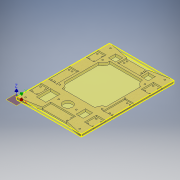
# Autodesk Inventor part: 3枚目
Saved by Autodesk Inventor 2018 (Build 220112000, 112)
## iProperties
Created: 2018-08-16
Part Number: 3枚目
Material: MDF 中密度繊維ボード
Document SubType Name: Modeling
Designer: shun2
Density: 0.8 g/cm^3
Appearance: ダンボール - 段ボール紙
Author: shun2
Autodesk Inventor part; units mm, degrees
ref_plane "YZ Plane" through (0, 0, 0) normal (1, 0, 0) x (0, 1, 0)
ref_plane "XZ Plane" through (0, 0, 0) normal (0, 1, 0) x (-1, 0, 0)
ref_plane "XY Plane" through (0, 0, 0) normal (0, 0, 1) x (1, 0, 0)
ref_plane "作業平面1" through (0, 0, 5.5) normal (0, 0, 1) x (1, 0, 0)
ref_plane "作業平面6" through (0, 0, 5.5) normal (0, 0, 1) x (1, 0, 0)
ref_plane "作業平面7" through (0, 0, 5.5) normal (0, 0, -1) x (-1, 0, 0)
sketch "スケッチ9" plane through (0, 0, 5.5) normal (0, 0, -1) x (-1, 0, 0)
  circle A0 centre (-11, 186.7239) radius 1.6
  circle A1 centre (-11, 8) radius 1.6
  line L0 (-6.4, 186.7239) -> (-15.6, 186.7239)
  line L1 (-6.4, 8) -> (-15.6, 8)
  line L2 (-98, 8) -> (-133, 0)
  line L3 (-46.1667, 8) -> (-3, 0)
  line L4 (0, 0) -> (-3, 0)
  line L5 (-3.0456, 195.0736) -> (-45.187, 186.7239)
  line L6 (-132.9544, 195.0736) -> (-90.813, 186.7239)
  line L7 (-129.6, 186.7239) -> (-120.4, 186.7239)
  circle A2 centre (-125, 186.7239) radius 1.6
  line L8 (-129.6, 8) -> (-120.4, 8)
  circle A3 centre (-125, 8) radius 1.6
  line L9 (-133, 0) -> (-136, 0)
  line L10 (0, 195.0736) -> (-3.0456, 195.0736)
  line L11 (-132.9544, 195.0736) -> (-136, 195.0736)
  line L12 (0, 195.0736) -> (0, 0)
  line L13 (-136, 0) -> (-136, 195.0736)
  line L14 (-90.813, 186.7239) -> (-45.187, 186.7239)
  line L15 (-98, 8) -> (-46.1667, 8)
  point P0 (0, 0)
  constraints: 32 end point, 4 centre point, 4 horizontal, 2 parallel, 1 perpendicular, 1 vertical
extrude "押し出し9" add sketch "スケッチ9" against normal blind 5.5
ref_plane "作業平面8" through (0, 0, 5.5) normal (0, 0, -1) x (-1, 0, 0)
sketch "スケッチ10" plane through (0, 0, 5.5) normal (0, 0, -1) x (-1, 0, 0)
  line L0 (0, 0) -> (0, 225.6064) construction
  circle A0 centre (-68, 39.7463) radius 10
  dimension "d399" = 20
  constraints: 2 end point, 1 centre point, 1 vertical, 1 other
  measures "d399" diameter of A0
extrude "押し出し10" cut sketch "スケッチ10" against normal blind 5.5
sketch "スケッチ13" plane through (0, 0, 11) normal (0, 0, 1) x (1, 0, 0)
  line L0 (117, 65.5) -> (117, 111.126)
  line L1 (117, 65.5) -> (136, 65.5)
  line L2 (136, 111.126) -> (136, 65.5)
  line L3 (117, 111.126) -> (136, 111.126)
  line L4 (19, 65.5) -> (19, 111.126)
  line L5 (19, 65.5) -> (0, 65.5)
  line L6 (0, 111.126) -> (0, 65.5)
  line L7 (19, 111.126) -> (0, 111.126)
  line L8 (0, 40.5) -> (18.3, 40.5) projected
  line L9 (117.7, 40.5) -> (136, 40.5) projected
  line L10 (90.813, 186.7239) -> (45.187, 186.7239) projected
  line L11 (45.187, 186.7239) -> (90.813, 186.7239)
  line L12 (90.813, 186.7239) -> (90.813, 167.7239)
  line L13 (90.813, 167.7239) -> (45.187, 167.7239)
  line L14 (45.187, 167.7239) -> (45.187, 186.7239)
  line L15 (136, 0) -> (136, 195.0736) projected
  line L16 (0, 195.0736) -> (0, 0) projected
  point P0 (105.9625, 75.6175)
  point P1 (244.1196, 130.8174)
  point P2 (0, 62.936)
  point P3 (121.3594, 75.6175)
  point P4 (30.0375, 75.6175)
  point P5 (14.6406, 75.6175)
  dimension "d207" = 45.626
  dimension "d297" = 19
  dimension "d299" = 45.626
  dimension "d300" = 19
  dimension "d394" = 25
  dimension "d395" = 25
  dimension "d428" = 19
  dimension "d458" = 45.626
  constraints: 24 end point, 2 collinear, 2 parallel, 1 horizontal, 1 perpendicular
  measures "d207" distance between parallel lines of L3 L1
  measures "d297" distance between parallel lines of L0 L2
  measures "d299" distance between parallel lines of L7 L5
  measures "d300" distance between parallel lines of L6 L4
  measures "d394" distance between parallel lines of L5 L8
  measures "d395" distance between parallel lines of L1 L9
  measures "d428" distance of L11.end L12.end
  measures "d458" distance between parallel lines of L14 L12
extrude "押し出し13" cut sketch "スケッチ13" against normal blind 2.5
sketch "スケッチ14" plane through (132, 67.436, 11) normal (0, 0, 1) x (1, 0, 0)
  circle A0 centre (0, 39.19) radius 1.6
  line L0 (-15, 43.69) -> (4, 43.69) projected
  circle A1 centre (-6, 39.19) radius 1.6
  circle A2 centre (-6, 2.564) radius 1.6
  line L1 (4, -1.936) -> (-15, -1.936) projected
  circle A3 centre (0, 2.564) radius 1.6
  line L2 (-132, -18.936) -> (-132, 78.7879) projected
  line L3 (-132, 60.7739) -> (4.0811, 60.7739)
  line L4 (4.0811, 60.7739) -> (-63.9594, 60.7739)
  line L5 (-63.9594, 60.7739) -> (-63.9594, 40.19)
  circle A4 centre (-127.9189, 39.19) radius 1.6
  circle A5 centre (-121.9189, 39.19) radius 1.6
  circle A6 centre (-121.9189, 2.564) radius 1.6
  circle A7 centre (-127.9189, 2.564) radius 1.6
  line L6 (4, 28.69) -> (4, -16.936) projected
  circle A8 centre (-82.313, 115.288) radius 1.6
  line L7 (-86.813, 100.2879) -> (-86.813, 119.2879) projected
  circle A9 centre (-82.313, 109.288) radius 1.6
  circle A10 centre (-45.687, 115.288) radius 1.6
  line L8 (-41.187, 119.2879) -> (-41.187, 100.2879) projected
  circle A11 centre (-45.687, 109.288) radius 1.6
  point P0 (-132.5, -84.3342)
  dimension "d261" = 3.2
  dimension "d263" = 4.5
  dimension "d264" = 3.2
  dimension "d266" = 3.2
  dimension "d268" = 4.5
  dimension "d269" = 3.2
  dimension "d309" = 6
  dimension "d310" = 6
  dimension "d311" = 4
  dimension "d312" = 4
  dimension "d322" = 4.5
  dimension "d451" = 3.2
  dimension "d452" = 4.5
  dimension "d453" = 3.2
  dimension "d454" = 6
  dimension "d455" = 3.2
  dimension "d456" = 4.5
  dimension "d457" = 3.2
  constraints: 12 centre point, 6 end point, 4 symmetric about line, 1 horizontal, 1 midpoint, 1 point on line, 1 vertical, 6 other
  measures "d261" diameter of A0
  measures "d264" diameter of A1
  measures "d266" diameter of A2
  measures "d269" diameter of A3
  measures "d309" distance of A2.centre A3.centre
  measures "d310" distance of A1.centre A0.centre
  measures "d311" distance from line of L6 A3.centre
  measures "d312" distance from line of L6 A0.centre
  measures "d451" diameter of A8
  measures "d452" distance from line of L7 A8.centre
  measures "d453" diameter of A9
  measures "d454" distance of A8.centre A9.centre
  measures "d455" diameter of A10
  measures "d456" distance from line of A10.centre L8
  measures "d457" diameter of A11
extrude "押し出し14" cut sketch "スケッチ14" against normal blind 5.5
sketch "スケッチ15" plane through (0, 0, 5.5) normal (0, 0, -1) x (-1, 0, 0)
  circle A0 centre (-86.313, 182.724) radius 1.6 projected
  circle A1 centre (-49.687, 182.724) radius 1.6 projected
  circle A2 centre (-10.0811, 106.626) radius 1.6 projected
  circle A3 centre (-10.0811, 70) radius 1.6 projected
  circle A4 centre (-126, 70) radius 1.6 projected
  circle A5 centre (-132, 106.626) radius 1.6 projected
  circle A6 centre (-126, 106.626) radius 1.6 projected
  circle A7 centre (-132, 70) radius 1.6 projected
  circle A8 centre (-4.0811, 70) radius 1.6 projected
  circle A9 centre (-4.0811, 106.626) radius 1.6 projected
  circle A10 centre (-49.687, 176.724) radius 1.6 projected
  circle A11 centre (-86.313, 176.724) radius 1.6 projected
  circle A12 centre (-68, 39.7463) radius 10 projected
  circle A13 centre (-125, 186.7239) radius 1.6 projected
  circle A14 centre (-125, 8) radius 1.6 projected
  circle A15 centre (-11, 8) radius 1.6 projected
  circle A16 centre (-11, 186.7239) radius 1.6 projected
  line L0 (0, 0) -> (-3, 0) projected
  line L1 (0, 195.0736) -> (0, 0) projected
  line L2 (-3.0456, 195.0736) -> (0, 195.0736) projected
  line L3 (-45.187, 186.7239) -> (-3.0456, 195.0736) projected
  line L4 (-90.813, 186.7239) -> (-45.187, 186.7239) projected
  line L5 (-132.9544, 195.0736) -> (-90.813, 186.7239) projected
  line L6 (-136, 195.0736) -> (-132.9544, 195.0736) projected
  line L7 (-136, 0) -> (-136, 195.0736) projected
  line L8 (-133, 0) -> (-136, 0) projected
  line L9 (-98, 8) -> (-133, 0) projected
  line L10 (-46.1667, 8) -> (-98, 8) projected
  line L11 (-3, 0) -> (-46.1667, 8) projected
  line L12 (-68, 157.5716) -> (-68, 90.4161)
  circle A17 centre (-23.55, 157.5716) radius 1.6
  circle A18 centre (-23.55, 67.4016) radius 1.6
  line L13 (-33.55, 162.5716) -> (-68, 162.5716)
  line L14 (-33.55, 62.4016) -> (-68, 62.4016)
  arc A19 (-33.55, 162.5716) -> (-23.55, 148.4295) centre (-18.55, 162.5716) ccw
  arc A20 (-4.9029, 68.6272) -> (-5.6778, 70.1028) centre (-18.55, 62.4016) ccw
  arc A21 (-23.55, 76.5438) -> (-33.55, 62.4016) centre (-18.55, 62.4016) ccw
  line L15 (-23.55, 148.4295) -> (-23.55, 76.5438)
  circle A22 centre (-112.45, 157.5716) radius 1.6
  circle A23 centre (-112.45, 67.4016) radius 1.6
  line L16 (-102.45, 162.5716) -> (-68, 162.5716)
  line L17 (-102.45, 62.4016) -> (-68, 62.4016)
  arc A24 (-112.45, 148.4295) -> (-102.45, 162.5716) centre (-117.45, 162.5716) ccw
  arc A25 (-102.45, 62.4016) -> (-112.45, 76.5438) centre (-117.45, 62.4016) ccw
  line L18 (-112.45, 148.4295) -> (-112.45, 76.5438)
  constraints: 14 end point, 12 point on circle, 9 centre point, 8 symmetric about line, 1 perpendicular, 1 vertical, 4 other
extrude "押し出し16" cut sketch "スケッチ15" against normal blind 5.5 contours A17 | A18 | A19 L15 A21 L14 L17 A25 L18 A24 L16 L13 | A22 | A23
sketch "スケッチ16" plane through (0, 0, 11) normal (0, 0, 1) x (1, 0, 0)
  point P0 (0, 0)
sketch "スケッチ17" plane through (0, 0, 11) normal (0, 0, 1) x (1, 0, 0)
  line L0 (117, 111.126) -> (136, 111.126) projected
  line L1 (132.9544, 195.0736) -> (90.813, 186.7239) projected
  line L2 (45.187, 186.7239) -> (3.0456, 195.0736) projected
  line L3 (0, 111.126) -> (19, 111.126) projected
  line L4 (19, 111.126) -> (19, 65.5) projected
  line L5 (19, 65.5) -> (0, 65.5) projected
  line L6 (0, 0) -> (3, 0) projected
  line L7 (3, 0) -> (46.1667, 8) projected
  line L8 (98, 8) -> (133, 0) projected
  line L9 (136, 65.5) -> (117, 65.5) projected
  line L10 (117, 65.5) -> (117, 111.126) projected
  circle A0 centre (11, 8) radius 1.6 projected
  circle A1 centre (11, 186.7239) radius 1.6 projected
  circle A2 centre (45.187, 168.4239) radius 1
  circle A3 centre (90.813, 168.4239) radius 1
  line L11 (117, 65.5) -> (117, 111.126) projected
  circle A4 centre (117, 111.126) radius 1
  circle A5 centre (117, 65.5) radius 1
  line L12 (19, 111.126) -> (19, 65.5) projected
  circle A6 centre (19, 65.5) radius 1
  circle A7 centre (19, 111.126) radius 1
  line L13 (136, 195.0736) -> (132.9544, 195.0736) projected
  line L14 (3.0456, 195.0736) -> (0, 195.0736) projected
  line L15 (133, 0) -> (136, 0) projected
  line L16 (136, 111.126) -> (136, 195.0736) projected
  line L17 (0, 195.0736) -> (0, 111.126) projected
  line L18 (0, 65.5) -> (0, 0) projected
  line L19 (46.1667, 8) -> (98, 8) projected
  line L20 (136, 0) -> (136, 65.5) projected
  line L21 (90.813, 186.7239) -> (90.813, 167.7239) projected
  line L22 (90.813, 167.7239) -> (45.187, 167.7239) projected
  line L23 (45.187, 167.7239) -> (45.187, 186.7239) projected
  point P0 (0, 0)
  point P1 (117.7, 180.074)
  point P2 (18.3, 180.074)
  point P3 (18.3, 154.574)
  dimension "d372" = 2
  dimension "d373" = 2
  dimension "d376" = 2
  dimension "d393" = 2
  dimension "d416" = 2
  dimension "d417" = 2
  constraints: 6 centre point, 4 coincident
  measures "d372" diameter of A2
  measures "d373" diameter of A3
  measures "d376" diameter of A4
  measures "d393" diameter of A7
  measures "d416" diameter of A5
  measures "d417" diameter of A6
extrude "押し出し17" cut sketch "スケッチ17" against normal blind 3 contours L10 A4 L0 | L0 A4 L10 | A5 L9 L10 | L10 L9 A5 | L21 L22 A3 | A3 L22 L21 | L22 L23 A2 | A2 L23 L22 | A6 L4 L5 | L5 L4 A6 | A7 L4 L3 | L3 L4 A7
sketch "スケッチ19" plane through (0, 0, 11) normal (0, 0, 1) x (1, 0, 0)
  circle A0 centre (86.5945, 39.2943) radius 1.6
  circle A1 centre (49.4055, 39.2943) radius 1.6
  circle A2 centre (68, 39.7463) radius 10 projected
  point P0 (0, 0)
  dimension "d418" = 3.2
  dimension "d419" = 3.2
  dimension "d420" = 18.5945
  dimension "d421" = 18.5945
  constraints: 2 centre point
  measures "d418" diameter of A0
  measures "d419" diameter of A1
  measures "d420" horizontal distance of A2.centre A0.centre
  measures "d421" horizontal distance of A2.centre A1.centre
extrude "押し出し19" cut sketch "スケッチ19" against normal blind 10 contours A0 | A1
sketch "スケッチ21" plane through (0, 0, 11) normal (0, 0, 1) x (1, 0, 0)
  line L0 (0, 195.0736) -> (0, 0) projected
  line L1 (18.3, 25) -> (18.3, 50.5) projected
  line L2 (0, 25) -> (18.3, 25)
  line L3 (18.3, 25) -> (18.3, 50.5)
  line L4 (18.3, 50.5) -> (0, 50.5)
  line L5 (0, 50.5) -> (0, 25)
  line L6 (18.3, 170.074) -> (0, 170.074) projected
  line L7 (0, 170.074) -> (18.3, 170.074)
  line L8 (18.3, 170.074) -> (18.3, 144.574)
  line L9 (18.3, 144.574) -> (0, 144.574)
  line L10 (0, 144.574) -> (0, 170.074)
  line L11 (136, 170.074) -> (117.7, 170.074) projected
  line L12 (136, 144.574) -> (117.7, 144.574)
  line L13 (117.7, 144.574) -> (117.7, 170.074)
  line L14 (117.7, 170.074) -> (136, 170.074)
  line L15 (136, 170.074) -> (136, 144.574)
  line L16 (136, 25) -> (136, 50.5) projected
  line L17 (136, 25) -> (117.7, 25)
  line L18 (117.7, 25) -> (117.7, 50.5)
  line L19 (117.7, 50.5) -> (136, 50.5)
  line L20 (136, 50.5) -> (136, 25)
  line L21 (98, 8) -> (133, 0) projected
  line L22 (46.1667, 26.3) -> (46.1667, 8) projected
  line L23 (98, 8) -> (46.1667, 8)
  line L24 (46.1667, 8) -> (46.1667, 26.3)
  line L25 (46.1667, 26.3) -> (98, 26.3)
  line L26 (98, 26.3) -> (98, 8)
  dimension "d427" = 25.5
  constraints: 40 end point, 10 parallel, 5 horizontal, 5 perpendicular, 2 point on line
  measures "d427" distance of L7.end L8.end
sketch "スケッチ22" plane through (0, 0, 11) normal (0, 0, 1) x (1, 0, 0)
  circle A0 centre (4, 29) radius 1.6 projected
  circle A1 centre (4, 29) radius 1.6
  circle A2 centre (14.8, 29) radius 1.6 projected
  circle A3 centre (14.8, 29) radius 1.6
  circle A4 centre (14.8, 46.5) radius 1.6 projected
  circle A5 centre (14.8, 46.5) radius 1.6
  circle A6 centre (4, 46.5) radius 1.6 projected
  circle A7 centre (4, 46.5) radius 1.6
  circle A8 centre (121.2, 29) radius 1.6 projected
  circle A9 centre (121.2, 29) radius 1.6
  circle A10 centre (121.2, 46.5) radius 1.6
  circle A11 centre (131.9446, 29) radius 1.6
  circle A12 centre (131.9446, 46.5) radius 1.6
  circle A13 centre (132, 148.574) radius 1.6 projected
  circle A14 centre (132, 148.574) radius 1.6
  circle A15 centre (121.2, 148.574) radius 1.6
  circle A16 centre (132, 166.074) radius 1.6 projected
  circle A17 centre (132, 166.074) radius 1.6
  circle A18 centre (121.2, 166.074) radius 1.6 projected
  circle A19 centre (121.2, 166.074) radius 1.6
  circle A20 centre (4, 166.074) radius 1.6 projected
  circle A21 centre (4, 166.074) radius 1.6
  circle A22 centre (14.8, 166.074) radius 1.6 projected
  circle A23 centre (14.8, 166.074) radius 1.6
  circle A24 centre (14.8, 148.574) radius 1.6 projected
  circle A25 centre (14.8, 148.574) radius 1.6
  circle A26 centre (4, 148.574) radius 1.6 projected
  circle A27 centre (4, 148.574) radius 1.6
  circle A28 centre (94, 21.65) radius 1.6 projected
  circle A29 centre (94, 21.65) radius 1.6
  circle A30 centre (94, 12.65) radius 1.6 projected
  circle A31 centre (94, 12.65) radius 1.6
  point P0 (0, 0)
  dimension "d429" = 3.2
  dimension "d430" = 3.2
  dimension "d431" = 3.2
  dimension "d432" = 3.2
  dimension "d433" = 3.2
  dimension "d434" = 3.2
  dimension "d435" = 3.2
  dimension "d436" = 3.2
  dimension "d437" = 3.2
  dimension "d438" = 3.2
  dimension "d439" = 3.2
  dimension "d440" = 3.2
  dimension "d441" = 3.2
  dimension "d442" = 3.2
  dimension "d443" = 3.2
  dimension "d444" = 3.2
  dimension "d445" = 3.2
  dimension "d446" = 3.2
  constraints: 18 centre point, 14 coincident
  measures "d429" diameter of A1
  measures "d430" diameter of A3
  measures "d431" diameter of A5
  measures "d432" diameter of A7
  measures "d433" diameter of A9
  measures "d434" diameter of A10
  measures "d435" diameter of A11
  measures "d436" diameter of A12
  measures "d437" diameter of A14
  measures "d438" diameter of A15
  measures "d439" diameter of A17
  measures "d440" diameter of A19
  measures "d441" diameter of A21
  measures "d442" diameter of A23
  measures "d443" diameter of A25
  measures "d444" diameter of A27
  measures "d445" diameter of A29
  measures "d446" diameter of A31
extrude "押し出し20" cut sketch "スケッチ21" against normal blind 3
extrude "押し出し21" cut sketch "スケッチ22" against normal blind 10
sketch "スケッチ25" plane through (0, 0, 11) normal (0, 0, 1) x (1, 0, 0)
  line L0 (26.3, 50.5) -> (41.3, 50.5)
  line L1 (41.3, 50.5) -> (41.3, 20.5)
  line L2 (41.3, 20.5) -> (26.3, 20.5)
  line L3 (109.7, 50.5) -> (94.7, 50.5)
  line L4 (94.7, 50.5) -> (94.7, 30.5)
  line L5 (94.7, 30.5) -> (109.7, 30.5)
  line L6 (109.7, 30.5) -> (109.7, 50.5)
  line L7 (41.3, 167.1984) -> (26.3, 167.1984)
  line L8 (26.3, 167.1984) -> (26.3, 182.1984)
  line L9 (26.3, 182.1984) -> (41.3, 182.1984)
  line L10 (41.3, 182.1984) -> (41.3, 167.1984)
  line L11 (94.7, 167.1984) -> (109.7, 167.1984)
  line L12 (109.7, 167.1984) -> (109.7, 182.1984)
  line L13 (109.7, 182.1984) -> (94.7, 182.1984)
  line L14 (94.7, 182.1984) -> (94.7, 167.1984)
  line L15 (26.3, 20.5) -> (21.3, 20.5)
  line L16 (21.3, 20.5) -> (21.3, 50.5)
  line L17 (21.3, 50.5) -> (26.3, 50.5)
  line L18 (41.3, 50.5) -> (21.3, 50.5)
  line L19 (21.3, 50.5) -> (21.3, 20.5)
  line L20 (21.3, 20.5) -> (41.3, 20.5)
  line L21 (41.3, 20.5) -> (41.3, 50.5)
  point P0 (0, 0)
  dimension "d474" = 30
  dimension "d475" = 15
  dimension "d476" = 20
  dimension "d479" = 15
  dimension "d480" = 15
  dimension "d481" = 15
  dimension "d482" = 15
  constraints: 44 end point, 10 parallel, 7 horizontal, 6 perpendicular, 2 point on line
  measures "d474" distance of L0.end L1.end
  measures "d475" distance of L5.end L4.end
  measures "d476" distance of L4.end L3.end
  measures "d479" distance of L8.end L9.end
  measures "d480" distance of L7.end L8.end
  measures "d481" distance of L13.end L12.end
  measures "d482" distance of L12.end L11.end
extrude "押し出し22" cut sketch "スケッチ25" against normal blind 10
